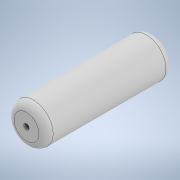
# Autodesk Inventor part: RubberHandleSleeveGBR
Saved by Autodesk Inventor 2020.1 (Build 241239000, 239)
## iProperties
Created: 2020-03-14
Part Number: RubberHandleSleeveGBR
Material: Generic
Document SubType Name: Modeling
Designer: super
Density: 1 g/cm^3
Appearance: Default
Author: super
Autodesk Inventor part; units mm, degrees
ref_plane "YZ Plane" through (0, 0, 0) normal (1, 0, 0) x (0, 1, 0)
ref_plane "XZ Plane" through (0, 0, 0) normal (0, 1, 0) x (-1, 0, 0)
ref_plane "XY Plane" through (0, 0, 0) normal (0, 0, 1) x (1, 0, 0)
sketch "Sketch1" plane through (0, 0, 0) normal (0, 1, 0) x (-1, 0, 0)
  line L0 (0, 0) -> (0, -113.5126)
  line L1 (0, -113.5126) -> (6.35, -113.5126)
  line L2 (6.35, -113.5126) -> (6.35, -3.9624)
  line L3 (0, 0) -> (15.0812, 0)
  line L4 (15.0812, 0) -> (15.0812, -3.9624)
  line L5 (15.0812, -3.9624) -> (6.35, -3.9624)
  line L6 (17.4625, -3.9624) -> (17.4625, -100.2955) construction
  dimension "d0" = 113.5126
  dimension "d1" = 6.35
  dimension "d2" = 109.5502
  dimension "d3" = 15.0813
  dimension "d4" = 2.3813
  constraints: 14 end point, 3 perpendicular, 1 horizontal, 1 parallel, 1 vertical
  measures "d0" distance of L0.start L0.end
  measures "d1" distance of L0.end L1.end
  measures "d2" distance of L1.end L2.end
  measures "d3" distance of L0.start L3.end
  measures "d4" distance of L4.end L6.start
revolve "Revolution1" add sketch "Sketch1" angle 360 about axis through (-17.4625, 0, -3.9624) along (0, 0, -1)
fillet "Fillet1" radius 6.35 2 edges at (-34.925, 0, -113.5126) (-34.925, 0, 0)
body "Solid1"
